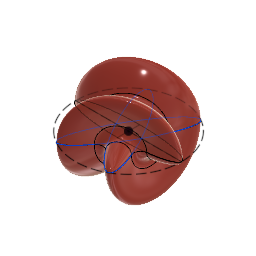
Atom Bomb Elliptic Star Hexasphericon (Autodesk Fusion 360 design; units mm, degrees)
Autodesk Fusion 360 part; units mm, degrees
sketch "Profile 3 ellipses" plane through (0, 0, 0) normal (0, 0, 1) x (1, 0, 0)
  circle A0 centre (0, 0) radius 30 construction
  ellipse E0 centre (0, 0) end of major axis (30, 0) minor radius 6.2761
  line L0 (-30, 0) -> (30, 0)
  line L1 (0, -6.2761) -> (0, 6.2761)
  ellipse E1 centre (0, 0) end of major axis (-15, 25.9808) minor radius 6.2761
  ellipse E2 centre (0, 0) end of major axis (-15, -25.9808) minor radius 6.2761
  line L2 (-30, 0) -> (30, 0)
  dimension "d1" = 60
  dimension "d3" = 360
  measures "d1" diameter of A0
revolve "Revolve1" add sketch "Profile 3 ellipses" angle 360 about axis through (-30, 0, 0) along (1, 0, 0) contours E0 L0 E2 L2 | E0 E1 E2 | E0 E1 E2 | E0 L0 L1 E1 L2 | E0 E1 E2 | E0 E1 E2 | E0 L0 L1 E2 L2 | E0 E1 E2 | E0 L0 E1 L2 picked at (20.3901, 1.2575) picked at (7.051, 4.0709) picked at (8.9619, 13.1308) picked at (2.1088, 3.6525) picked at (0, 8.1418) picked at (-6.5887, 13.8656) picked at (-2.1088, 3.6525) picked at (-7.051, 4.0709) picked at (-19.2537, 1.5231) makes body 1
split "Split1" by plane through (0, 0, 0) normal (0, 0, 1) bodies 1 makes body 2 at (4.5061, -17.5626, 3.5504)
fillet "Fillet1" radius 4 6 edges at (10.2202, 0, -5.9006) (0, 0, -11.8013) (-10.2202, 0, -5.9006) (0, 0, 11.8013) (-10.2202, 0, 5.9006) (10.2202, 0, 5.9006) on bodies 1 2
move_body "Move5" bodies 2 to x (0.5, -0.866025, 0) y (0.866025, 0.5, 0) z (0, 0, 1) at (0, 0, 0)
sketch "Magnet and pin holes" plane through (0, 0, 0) normal (0, 0, 1) x (1, 0, 0)
  circle A0 centre (0, 0) radius 5.4283
  circle A1 centre (0, 0) radius 12.5 construction
  circle A2 centre (-12.5, 0) radius 2.65
  circle A3 centre (-6.25, -10.8253) radius 2.65
  circle A4 centre (6.25, -10.8253) radius 2.65
  circle A5 centre (12.5, 0) radius 2.65
  circle A6 centre (6.25, 10.8253) radius 2.65
  circle A7 centre (-6.25, 10.8253) radius 2.65
  circle A8 centre (0, 0) radius 5.2
  dimension "d18" = 10.8567
  dimension "d19" = 25
  dimension "d20" = 5.3
  dimension "d22" = 360
  dimension "d29" = 10.4
  measures "d18" diameter of A0
  measures "d19" diameter of A1
  measures "d20" diameter of A2
  measures "d29" diameter of A8
extrude "Extrude1" cut sketch "Magnet and pin holes" along normal blind 4.5 contours A2 | A3 | A4 | A5 | A6 | A7 bodies 2
chamfer "Chamfer1" distance 2 angle 45 6 edges at (-14.9707, -0.9583, 4.5) (-8.7207, -11.7836, 4.5) (3.7793, -11.7836, 4.5) (-8.7207, 9.867, 4.5) (10.0293, -0.9583, 4.5) (3.7793, 9.867, 4.5) on bodies 2
extrude "Extrude2" cut sketch "Magnet and pin holes" along normal blind 10 contours A0 | A8 bodies 2
chamfer "Chamfer2" distance 2 angle 45 1 edges at (-5.061, -1.963, 10) on bodies 2
extrude "Extrude3" add sketch "Magnet and pin holes" along normal mid plane 19 separate body contours A8 makes body 3
chamfer "Chamfer3" distance 2.5 angle 45 2 edges at (-4.8481, -1.8804, 9.5) (-4.8481, 1.8804, -9.5) on bodies 3
named bodies: "Bottom", "Top", "Peg"
